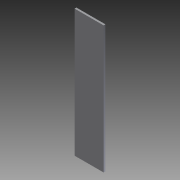
# Autodesk Inventor part: side
Saved by Autodesk Inventor 2011 (Build 150239000, 239)
## iProperties
Created: 2011-10-08
Part Number: side
Document SubType Name: Modeling
Designer: Matthew
Density: 1 g/cm^3
Author: Matthew
Autodesk Inventor part; units mm, degrees
ref_plane "YZ Plane" through (0, 0, 0) normal (1, 0, 0) x (0, 1, 0)
ref_plane "XZ Plane" through (0, 0, 0) normal (0, 1, 0) x (-1, 0, 0)
ref_plane "XY Plane" through (0, 0, 0) normal (0, 0, 1) x (1, 0, 0)
sketch "Sketch1" plane through (0, 0, 0) normal (0, 0, 1) x (1, 0, 0)
  line L0 (-22.2985, 25.8576) -> (117.4015, 25.8576)
  line L1 (117.4015, 25.8576) -> (117.4015, -278.9424)
  line L2 (117.4015, -278.9424) -> (-22.2985, -278.9424)
  line L3 (-22.2985, -278.9424) -> (-22.2985, 25.8576)
  point P0 (0, 0)
  dimension "d0" = 139.7
  dimension "d1" = 304.8
  constraints: 8 end point, 2 parallel, 1 horizontal, 1 perpendicular
  measures "d0" distance of L1.end L2.end
  measures "d1" distance of L0.end L1.end
extrude "Extrusion1" add sketch "Sketch1" along normal blind 6.35
sketch "Sketch2" plane through (117.4015, -278.9424, 0) normal (1, 0, 0) x (0, 0, -1)
  line L0 (-6.35, 304.8) -> (-6.35, 0) projected
  line L1 (0, 0) -> (-6.35, 0) projected
  line L2 (0, 304.8) -> (0, 0) projected
  line L3 (0, 304.8) -> (-6.35, 304.8) projected
  point P0 (0, 278.9424)
extrude "Extrusion2" add sketch "Sketch2" along normal blind 12.7
sketch "Sketch3" plane through (130.1015, -278.9424, 0) normal (1, 0, 0) x (0, 0, -1)
  line L0 (-6.35, 304.8) -> (0, 304.8) projected
  line L1 (-6.35, 0) -> (-6.35, 304.8) projected
  line L2 (0, 0) -> (-6.35, 0) projected
  line L3 (0, 304.8) -> (0, 0) projected
  point P0 (0, 278.9424)
extrude "Extrusion3" cut sketch "Sketch3" against normal blind 12.7
sketch "Sketch4" plane through (117.4015, -278.9424, 0) normal (1, 0, 0) x (0, 0, -1)
  line L0 (-6.35, 0) -> (-6.35, 304.8) projected
  line L1 (0, 0) -> (-6.35, 0) projected
  line L2 (0, 304.8) -> (0, 0) projected
  line L3 (-6.35, 304.8) -> (0, 304.8) projected
  point P0 (0, 278.9424)
extrude "Extrusion4" cut sketch "Sketch4" against normal blind 38.1
sketch "Sketch5" plane through (0, 0, 0) normal (0, 0, -1) x (-1, 0, 0)
  line L0 (-79.3015, -278.9424) -> (22.2985, -278.9424)
  line L1 (22.2985, -278.9424) -> (22.2985, -532.9424)
  line L2 (22.2985, -532.9424) -> (-79.3015, -532.9424)
  line L3 (-79.3015, -532.9424) -> (-79.3015, -278.9424)
  point P0 (0, 0)
  dimension "d10" = 254
  constraints: 8 end point, 2 parallel, 1 horizontal, 1 perpendicular
  measures "d10" distance of L0.end L1.end
extrude "Extrusion5" add sketch "Sketch5" against normal blind 6.35
sketch "Sketch6" plane through (-22.2985, -532.9424, 0) normal (0, -1, 0) x (1, 0, 0)
  line L0 (101.6, 6.35) -> (0, 6.35) projected
  line L1 (0, 0) -> (0, 6.35) projected
  line L2 (101.6, 0) -> (0, 0) projected
  line L3 (101.6, 0) -> (101.6, 6.35) projected
  point P0 (22.2985, 0)
extrude "Extrusion6" cut sketch "Sketch6" against normal blind 127
sketch "Sketch7" plane through (-22.2985, 25.8576, 6.35) normal (0, 1, 0) x (1, 0, 0)
  line L0 (101.6, 0) -> (101.6, 6.35) projected
  line L1 (0, 6.35) -> (101.6, 6.35) projected
  line L2 (0, 6.35) -> (0, 0) projected
  line L3 (0, 0) -> (101.6, 0) projected
  point P0 (22.2985, 6.35)
extrude "Extrusion7" add sketch "Sketch7" along normal blind 12.7
sketch "Sketch8" plane through (0, 0, 6.35) normal (0, 0, 1) x (1, 0, 0)
  line L0 (-22.2985, -405.9424) -> (79.3015, -405.9424) projected
  line L1 (79.3015, -405.9424) -> (79.3015, 38.5576) projected
  line L2 (-22.2985, -405.9424) -> (-22.2985, 38.5576) projected
  line L3 (79.3015, -405.9424) -> (79.3015, -386.8924)
  line L4 (79.3015, -386.8924) -> (-22.2985, -386.8924)
  point P0 (0, 0)
  dimension "d17" = 19.05
  constraints: 4 end point, 2 point on line, 1 perpendicular
  measures "d17" distance of L0.end L3.end
extrude "Extrusion8" cut sketch "Sketch8" against normal blind 25.4
sketch "Sketch9" plane through (0, 0, 6.35) normal (0, 0, 1) x (1, 0, 0)
  line L0 (79.3015, -386.8924) -> (79.3015, 38.5576) projected
  line L1 (-22.2985, 38.5576) -> (79.3015, 38.5576)
  line L2 (79.3015, 38.5576) -> (79.3015, 32.2076)
  line L3 (79.3015, 32.2076) -> (-22.2985, 32.2076)
  line L4 (-22.2985, 32.2076) -> (-22.2985, 38.5576)
  point P0 (0, 0)
  dimension "d20" = 6.35
  constraints: 8 end point, 2 parallel, 1 horizontal, 1 perpendicular, 1 point on line
  measures "d20" distance of L1.end L2.end
extrude "Extrusion9" cut sketch "Sketch9" against normal blind 25.4
body "Solid1"
